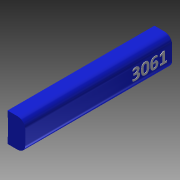
# Autodesk Inventor part: Bumper Cover Part1 (26x28 robot)
Saved by Autodesk Inventor 2013 (Build 170138000, 138)
## iProperties
Created: 2013-01-06
Part Number: Bumper Cover Part1 (26x28 robot)
Material: Generic
Document SubType Name: Modeling
Designer: Moses
Density: 1 g/cm^3
Mass: 359.1 g
Surface Area: 4483.46 cm^2
Volume: 359.1 cm^3
Author: Moses
Autodesk Inventor part; units mm, degrees
ref_plane "YZ Plane" through (0, 0, 0) normal (1, 0, 0) x (0, 1, 0)
ref_plane "XZ Plane" through (0, 0, 0) normal (0, 1, 0) x (-1, 0, 0)
ref_plane "XY Plane" through (0, 0, 0) normal (0, 0, 1) x (1, 0, 0)
sketch "Sketch1" plane through (0, 0, 0) normal (0, 0, 1) x (1, 0, 0)
  line L0 (-6.35, 63.5) -> (-6.35, -63.5) construction
  line L1 (6.35, 63.5) -> (-6.35, 63.5) construction
  line L2 (-6.35, -63.5) -> (6.35, -63.5) construction
  circle A0 centre (38.1, -31.75) radius 31.75 construction
  circle A1 centre (38.1, 31.75) radius 31.75 construction
  line L3 (6.35, 63.5) -> (38.1, 63.5) construction
  line L4 (69.85, 31.75) -> (69.85, -31.75) construction
  line L5 (6.35, -63.5) -> (38.1, -63.5) construction
  line L6 (38.1, 65.0875) -> (-7.9375, 65.0875)
  line L7 (-7.9375, -65.0875) -> (38.1, -65.0875)
  arc A2 (38.1, -65.0875) -> (71.4375, -31.75) centre (38.1, -31.75) ccw
  arc A3 (71.4375, 31.75) -> (38.1, 65.0875) centre (38.1, 31.75) ccw
  line L8 (71.4375, 31.75) -> (71.4375, -31.75)
  line L9 (38.1, 65.0875) -> (38.1, 63.5) construction
  arc A4 (69.85, 31.75) -> (38.1, 63.5) centre (38.1, 31.75) ccw
  arc A5 (38.1, -63.5) -> (69.85, -31.75) centre (38.1, -31.75) ccw
  line L10 (38.1, 63.5) -> (-6.35, 63.5)
  line L11 (38.1, -63.5) -> (-6.35, -63.5)
  line L12 (69.85, 31.75) -> (69.85, -31.75)
  line L13 (-6.35, 63.5) -> (-6.35, 38.1)
  line L14 (-6.35, 38.1) -> (-7.9375, 38.1)
  line L15 (-7.9375, 38.1) -> (-7.9375, 65.0875)
  line L16 (-7.9375, -65.0875) -> (-7.9375, -38.1)
  line L17 (-7.9375, -38.1) -> (-6.35, -38.1)
  line L18 (-6.35, -63.5) -> (-6.35, -38.1)
  line L19 (-6.35, 38.1) -> (-6.35, -38.1)
  point P0 (0, 0)
  point P1 (38.1, 64.2937)
  dimension "d3" = 25.4
  dimension "d5" = 1.5875
  dimension "d6" = 1.5875
  dimension "d7" = 25.4
  dimension "d9" = 1.5875
  constraints: 34 end point, 14 tangent, 12 point on circle, 6 perpendicular, 4 centre point, 3 collinear, 3 parallel, 2 coincident, 2 point on line, 1 concentric, 1 midpoint, 1 vertical
  measures "d3" distance of L0.start L13.end
  measures "d5" distance between parallel lines of L0 L15
  measures "d6" distance between parallel lines of L0 L16
  measures "d7" distance of L0.end L17.end
  measures "d9" distance of L6.start L3.end
extrude "Extrusion1" add sketch "Sketch1" along normal blind 1.5875
extrude "Extrusion2" add sketch "Sketch1" against normal blind 657.225 contours A3 L8 A2 L7 L16 L17 L18 L11 A5 L12 A4 L10 L13 L14 L15 L6
sketch "Sketch2" plane through (0, 0, -657.225) normal (0, 0, -1) x (-1, 0, 0)
  line L0 (-38.1, 63.5) -> (6.35, 63.5) projected
  line L1 (6.35, 63.5) -> (6.35, 38.1) projected
  line L2 (6.35, 38.1) -> (7.9375, 38.1) projected
  line L3 (7.9375, 38.1) -> (7.9375, 65.0875) projected
  line L4 (7.9375, 65.0875) -> (-38.1, 65.0875) projected
  arc A0 (-38.1, 65.0875) -> (-71.4375, 31.75) centre (-38.1, 31.75) ccw projected
  line L5 (-71.4375, 31.75) -> (-71.4375, -31.75) projected
  arc A1 (-71.4375, -31.75) -> (-38.1, -65.0875) centre (-38.1, -31.75) ccw projected
  line L6 (-38.1, -65.0875) -> (7.9375, -65.0875) projected
  line L7 (7.9375, -65.0875) -> (7.9375, -38.1) projected
  line L8 (7.9375, -38.1) -> (6.35, -38.1) projected
  line L9 (6.35, -38.1) -> (6.35, -63.5) projected
  line L10 (6.35, -63.5) -> (-38.1, -63.5) projected
  arc A2 (-69.85, -31.75) -> (-38.1, -63.5) centre (-38.1, -31.75) ccw projected
  line L11 (-69.85, -31.75) -> (-69.85, 31.75) projected
  arc A3 (-38.1, 63.5) -> (-69.85, 31.75) centre (-38.1, 31.75) ccw projected
  line L12 (6.35, 38.1) -> (6.35, -38.1)
  point P0 (0, 0)
  constraints: 2 end point, 1 parallel
extrude "Extrusion3" add sketch "Sketch2" along normal blind 1.5875
sketch "Sketch3" plane through (71.4375, -31.75, 1.5875) normal (1, 0, 0) x (0, 0, -1)
  line L0 (0, 0) -> (0, 63.5) projected
  line L1 (660.4, 63.5) -> (660.4, 0) projected
  line L2 (482.6, 63.5) -> (635, 63.5) construction
  line L3 (635, 63.5) -> (635, 0) construction
  line L4 (635, 0) -> (482.6, 0) construction
  line L5 (482.6, 0) -> (482.6, 63.5) construction
  line L6 (660.4, 31.75) -> (0, 31.75) construction
  spline S0 degree 2 poles (514.8687, 21.2561) (514.8687, 17.4878) (511.9591, 11.6208) (506.8075, 7.614) (499.6049, 5.563) (495.3596, 5.563) knots 0 0 0 1 2 3 4 4 4
  spline S1 degree 2 poles (495.3596, 5.563) (492.7839, 5.563) (488.2524, 6.3262) (484.7703, 7.3755) (482.4808, 8.568) (481.813, 9.1881) (481.4314, 9.999) (481.1452, 11.0484) (481.0498, 12.6225) (481.0498, 13.7673) knots 0 0 0 1 2 3 4 5 6 7 8 8 8
  spline S2 degree 2 poles (481.0498, 13.7673) (481.0498, 15.6753) (481.6699, 17.1062) (482.29, 17.1062) knots 0 0 0 1 2 2 2
  spline S3 degree 2 poles (482.29, 17.1062) (482.6716, 17.1062) (484.6272, 16.0569) (487.5846, 14.8167) (491.5914, 13.7673) (494.1194, 13.7673) knots 0 0 0 1 2 3 4 4 4
  spline S4 degree 2 poles (494.1194, 13.7673) (496.2659, 13.7673) (499.5572, 14.769) (501.8468, 16.6293) (502.9915, 19.2527) (502.9915, 20.8268) knots 0 0 0 1 2 3 4 4 4
  spline S5 degree 2 poles (502.9915, 20.8268) (502.9915, 22.5917) (501.6083, 25.406) (498.9371, 27.4093) (494.8349, 28.5064) (492.0207, 28.5064) knots 0 0 0 1 2 3 4 4 4
  line L7 (492.0207, 28.5064) -> (487.6323, 28.5064)
  spline S6 degree 2 poles (487.6323, 28.5064) (487.1553, 28.5064) (486.4398, 28.7926) (485.9628, 29.6512) (485.772, 31.1776) (485.772, 32.3701) knots 0 0 0 1 2 3 4 4 4
  spline S7 degree 2 poles (485.772, 32.3701) (485.772, 33.5149) (485.9628, 34.9459) (486.3921, 35.7091) (487.0599, 36.043) (487.5369, 36.043) knots 0 0 0 1 2 3 4 4 4
  line L8 (487.5369, 36.043) -> (491.973, 36.043)
  spline S8 degree 2 poles (491.973, 36.043) (494.2625, 36.043) (497.7923, 37.0923) (500.1773, 39.048) (501.4175, 41.8146) (501.4175, 43.5318) knots 0 0 0 1 2 3 4 4 4
  spline S9 degree 2 poles (501.4175, 43.5318) (501.4175, 44.8197) (500.5589, 47.1092) (498.8894, 48.7787) (496.2182, 49.7804) (494.4056, 49.7804) knots 0 0 0 1 2 3 4 4 4
  spline S10 degree 2 poles (494.4056, 49.7804) (492.3546, 49.7804) (488.7771, 48.5879) (485.9151, 47.1092) (483.9117, 45.8691) (483.4347, 45.8691) knots 0 0 0 1 2 3 4 4 4
  spline S11 degree 2 poles (483.4347, 45.8691) (483.1485, 45.8691) (482.6716, 46.1553) (482.3377, 46.9185) (482.1946, 48.3971) (482.1946, 49.5896) knots 0 0 0 1 2 3 4 4 4
  spline S12 degree 2 poles (482.1946, 49.5896) (482.1946, 50.5436) (482.29, 51.8315) (482.5285, 52.6901) (482.8623, 53.3102) (483.6255, 54.0734) (486.0582, 55.5521) (489.7311, 56.9831) (494.5487, 57.937) (497.363, 57.937) knots 0 0 0 1 2 3 4 5 6 7 8 8 8
  spline S13 degree 2 poles (497.363, 57.937) (501.0359, 57.937) (506.7121, 56.2199) (510.5758, 52.9763) (512.5792, 48.254) (512.5792, 45.249) knots 0 0 0 1 2 3 4 4 4
  spline S14 degree 2 poles (512.5792, 45.249) (512.5792, 42.9594) (511.3867, 39.0003) (509.1448, 35.8522) (505.7104, 33.658) (503.5162, 33.1333) knots 0 0 0 1 2 3 4 4 4
  line L9 (503.5162, 33.1333) -> (503.5162, 32.9902)
  spline S15 degree 2 poles (503.5162, 32.9902) (506.1397, 32.704) (510.385, 30.6052) (513.2946, 27.5047) (514.8687, 23.5457) (514.8687, 21.2561) knots 0 0 0 1 2 3 4 4 4
  spline S16 degree 2 poles (556.6535, 31.9408) (556.6535, 25.883) (554.6978, 16.1046) (550.2618, 9.2358) (543.2023, 5.563) (538.0984, 5.563) knots 0 0 0 1 2 3 4 4 4
  spline S17 degree 2 poles (538.0984, 5.563) (532.8992, 5.563) (526.0781, 9.1404) (522.1191, 15.8184) (520.4973, 25.4537) (520.4973, 31.5592) knots 0 0 0 1 2 3 4 4 4
  spline S18 degree 2 poles (520.4973, 31.5592) (520.4973, 37.5693) (522.5007, 47.3954) (526.889, 54.2642) (533.9962, 57.937) (539.0524, 57.937) knots 0 0 0 1 2 3 4 4 4
  spline S19 degree 2 poles (539.0524, 57.937) (544.2516, 57.937) (551.1204, 54.3596) (555.0794, 47.6816) (556.6535, 38.0463) (556.6535, 31.9408) knots 0 0 0 1 2 3 4 4 4
  spline S20 degree 2 poles (546.3027, 31.4638) (546.3027, 35.0413) (545.9211, 40.5744) (545.1102, 44.6289) (543.87, 47.4431) (542.1529, 49.1126) (539.9587, 49.8281) (538.6231, 49.8281) knots 0 0 0 1 2 3 4 5 6 6 6
  spline S21 degree 2 poles (538.6231, 49.8281) (536.3335, 49.8281) (533.3285, 47.5862) (531.5636, 43.1502) (530.8481, 36.4723) (530.8481, 32.0839) knots 0 0 0 1 2 3 4 4 4
  spline S22 degree 2 poles (530.8481, 32.0839) (530.8481, 26.6462) (531.7067, 19.5866) (533.5669, 15.3891) (536.4289, 13.7196) (538.48, 13.7196) knots 0 0 0 1 2 3 4 4 4
  spline S23 degree 2 poles (538.48, 13.7196) (540.0064, 13.7196) (542.3437, 14.7213) (544.1085, 16.6769) (545.301, 19.6343) (546.0165, 23.5457) (546.3027, 28.4587) (546.3027, 31.4638) knots 0 0 0 1 2 3 4 5 6 6 6
  spline S24 degree 2 poles (596.9596, 23.3549) (596.9596, 19.5389) (594.6223, 13.0041) (590.0909, 8.2818) (583.413, 5.563) (579.0723, 5.563) knots 0 0 0 1 2 3 4 4 4
  spline S25 degree 2 poles (579.0723, 5.563) (575.5902, 5.563) (570.3433, 7.1847) (566.5273, 10.1898) (564.0946, 14.4828) (562.616, 19.8728) (562.0913, 26.2169) (562.0913, 29.7466) knots 0 0 0 1 2 3 4 5 6 6 6
  spline S26 degree 2 poles (562.0913, 29.7466) (562.0913, 32.704) (562.6637, 39.1911) (564.3808, 45.4398) (567.4336, 51.116) (572.2036, 55.409) (579.0723, 57.8893) (583.7469, 57.8893) knots 0 0 0 1 2 3 4 5 6 6 6
  spline S27 degree 2 poles (583.7469, 57.8893) (585.2255, 57.8893) (588.2783, 57.5554) (590.8541, 56.9831) (592.619, 56.2676) (593.2391, 55.7906) (593.5253, 55.1705) (593.7161, 54.4073) (593.8115, 53.3102) (593.8115, 52.547) knots 0 0 0 1 2 3 4 5 6 7 8 8 8
  spline S28 degree 2 poles (593.8115, 52.547) (593.8115, 51.3068) (593.7161, 49.685) (593.3822, 48.8264) (592.8098, 48.3971) (592.4282, 48.3971) knots 0 0 0 1 2 3 4 4 4
  spline S29 degree 2 poles (592.4282, 48.3971) (591.9512, 48.3971) (590.4725, 48.9218) (588.3737, 49.5419) (585.5117, 50.0189) (583.6515, 50.0189) knots 0 0 0 1 2 3 4 4 4
  spline S30 degree 2 poles (583.6515, 50.0189) (580.4556, 50.0189) (576.0672, 47.6816) (573.3484, 43.6749) (572.1082, 38.3802) (572.0605, 35.4229) knots 0 0 0 1 2 3 4 4 4
  spline S31 degree 2 poles (572.0605, 35.4229) (572.9191, 35.9476) (575.1609, 37.0446) (577.7844, 37.8078) (580.7895, 38.3325) (582.5544, 38.3325) knots 0 0 0 1 2 3 4 4 4
  spline S32 degree 2 poles (582.5544, 38.3325) (586.3703, 38.3325) (591.8558, 36.2338) (595.3378, 32.3224) (596.9596, 26.7416) (596.9596, 23.3549) knots 0 0 0 1 2 3 4 4 4
  spline S33 degree 2 poles (586.895, 22.4009) (586.895, 24.3566) (586.1795, 27.4093) (584.6054, 29.4604) (582.0297, 30.5098) (580.2171, 30.5098) knots 0 0 0 1 2 3 4 4 4
  spline S34 degree 2 poles (580.2171, 30.5098) (579.12, 30.5098) (576.9735, 30.1282) (574.9701, 29.4127) (573.0622, 28.4587) (572.2513, 27.8863) knots 0 0 0 1 2 3 4 4 4
  spline S35 degree 2 poles (572.2513, 27.8863) (572.2513, 23.7365) (573.2053, 18.1079) (575.0178, 14.8644) (577.8321, 13.4811) (579.6447, 13.4811) knots 0 0 0 1 2 3 4 4 4
  spline S36 degree 2 poles (579.6447, 13.4811) (581.4573, 13.4811) (584.1761, 14.8167) (585.941, 17.2493) (586.895, 20.4929) (586.895, 22.4009) knots 0 0 0 1 2 3 4 4 4
  spline S37 degree 2 poles (636.264, 10.3806) (636.264, 9.2835) (636.0255, 7.7571) (635.5962, 6.8508) (635.0715, 6.4693) (634.69, 6.4693) knots 0 0 0 1 2 3 4 4 4
  line L10 (634.69, 6.4693) -> (606.7857, 6.4693)
  spline S38 degree 2 poles (606.7857, 6.4693) (606.4518, 6.4693) (605.9271, 6.8508) (605.4978, 7.7571) (605.2593, 9.2835) (605.2593, 10.3806) knots 0 0 0 1 2 3 4 4 4
  spline S39 degree 2 poles (605.2593, 10.3806) (605.2593, 11.4777) (605.4501, 13.0041) (605.8794, 13.9581) (606.4518, 14.3874) (606.7857, 14.3874) knots 0 0 0 1 2 3 4 4 4
  line L11 (606.7857, 14.3874) -> (616.1825, 14.3874)
  line L12 (616.1825, 14.3874) -> (616.1825, 47.3477)
  line L13 (616.1825, 47.3477) -> (608.0259, 42.864)
  spline S40 degree 2 poles (608.0259, 42.864) (607.1673, 42.4347) (606.0225, 42.2439) (605.3547, 42.9117) (605.1162, 44.5335) (605.1162, 46.0122) knots 0 0 0 1 2 3 4 4 4
  spline S41 degree 2 poles (605.1162, 46.0122) (605.1162, 46.9662) (605.2116, 48.1586) (605.4978, 49.0172) (606.0702, 49.5896) (606.5472, 49.8758) knots 0 0 0 1 2 3 4 4 4
  line L14 (606.5472, 49.8758) -> (617.375, 56.8877)
  spline S42 degree 2 poles (617.375, 56.8877) (617.6135, 57.0785) (618.1859, 57.2692) (619.1399, 57.3646) (620.6663, 57.4123) (621.8588, 57.4123) knots 0 0 0 1 2 3 4 4 4
  spline S43 degree 2 poles (621.8588, 57.4123) (623.3375, 57.4123) (625.1977, 57.3169) (626.104, 57.0308) (626.4379, 56.5538) (626.4379, 56.2199) knots 0 0 0 1 2 3 4 4 4
  line L15 (626.4379, 56.2199) -> (626.4379, 14.3874)
  line L16 (626.4379, 14.3874) -> (634.69, 14.3874)
  spline S44 degree 2 poles (634.69, 14.3874) (635.0715, 14.3874) (635.6439, 13.9581) (636.0732, 13.0041) (636.264, 11.4777) (636.264, 10.3806) knots 0 0 0 1 2 3 4 4 4
  point P0 (1.5875, 31.75)
  point P1 (635, 31.75)
  dimension "d41" = 25.4
  dimension "d42" = 152.4
  constraints: 3 midpoint, 2 end point, 2 point on line, 2 other
  measures "d41" distance between parallel lines of L1 L3
  measures "d42" distance between parallel lines of L3 L5
extrude "Extrusion5" add sketch "Sketch3" along normal blind 1.5875
body "Solid1"
